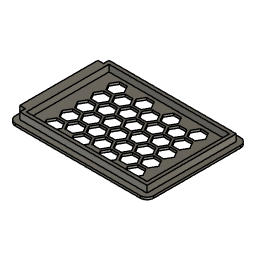
Mini-Amp Case V3 - Cover (Autodesk Fusion 360 design; units mm, degrees)
Autodesk Fusion 360 part; units mm, degrees
(part 1 of 2)
sketch "Sketch1" plane through (0, 0, 0) normal (0, 0, 1) x (1, 0, 0)
  line L0 (-1, -1) -> (57, -1)
  line L1 (57, -1) -> (57, 40)
  line L2 (57, 40) -> (-1, 40)
  line L3 (-1, 40) -> (-1, -1)
  line L4 (-3, -3) -> (59, -3)
  line L5 (59, -3) -> (59, 42)
  line L6 (59, 42) -> (-3, 42)
  line L7 (-3, 42) -> (-3, -3)
  constraint horizontal L0
  constraint vertical L1
  constraint horizontal L2
  constraint vertical L3
  constraint horizontal L4
  constraint vertical L5
  constraint horizontal L6
  constraint vertical L7
extrude "Extrude1" add sketch "Sketch1" along normal blind 3 contours L0 L1 L2 L3 | L4 L5 L6 L7
extrude "Extrude2" add sketch "Sketch1" along normal blind 21
sketch "Sketch2" plane through (59, 0, 0) normal (1, 0, 0) x (0, 1, 0)
  line L0 (-3, 0) -> (42, 0)
  line L1 (42, 0) -> (42, 21)
  line L2 (42, 21) -> (-3, 21)
  line L3 (-3, 21) -> (-3, 0)
  line L4 (42, 0) -> (42, 12.5) construction
  line L5 (42, 12.5) -> (27, 12.5) construction
  circle A0 centre (27, 12.5) radius 5
  dimension "d11" = 15
  dimension "d20" = 12.5
  constraint coincident L0.end L1.start
  constraint coincident L1 L4.end
  constraint perpendicular L0 L4
  constraint perpendicular L4 L5
  constraint coincident L5.end A0.centre
  measures "d11" distance of L1 L5.end
  measures "d20" distance of L0 L5.end
extrude "Extrude3" cut sketch "Sketch2" against normal blind 3 contours A0
sketch "Sketch3" plane through (-3, 0, 0) normal (-1, 0, 0) x (0, -1, 0)
  line L0 (-42, 0) -> (3, 0)
  line L1 (3, 0) -> (3, 21)
  line L2 (3, 21) -> (-42, 21)
  line L3 (-42, 21) -> (-42, 0)
  line L4 (-37, 7) -> (-37, 21)
  line L5 (-37, 21) -> (-2, 21)
  line L6 (-2, 21) -> (-2, 7)
  line L7 (-2, 7) -> (-37, 7)
  constraint perpendicular L0 L4
  constraint perpendicular L1 L5
  constraint perpendicular L5 L6
  constraint perpendicular L4 L7
  constraint coincident L2 L4.end
extrude "Extrude4" cut sketch "Sketch3" against normal blind 3 contours L2 L4 L5 L6 L7
fillet "Fillet1" radius 3 4 edges at (59, -3, 10.5) (59, 42, 10.5) (-3, 42, 10.5) (-3, -3, 10.5)
sketch "Sketch4" plane through (0, 0, 3) normal (0, 0, 1) x (-1, 0, 0)
  line L0 (1, 1) -> (-57, 1)
  line L1 (-57, 1) -> (-57, -40)
  line L2 (-57, -40) -> (1, -40)
  line L3 (1, -40) -> (1, 1)
  point P0 (-29.8405, -19.6761)
extrude "Extrude5" cut 1 faces at (37.3333, 12, 0) along direction (0, 0, 1) blind 1
sketch "Sketch5" plane through (0, 0, 3) normal (0, 0, 1) x (-1, 0, 0)
  line L0 (-8.2346, 0) -> (-7.3686, -1.5)
  line L1 (-7.3686, -1.5) -> (-5.0592, -1.5)
  line L2 (-5.0592, -1.5) -> (-4.1932, 0)
  line L3 (-0.7291, 0) -> (-3.0385, 0)
  line L4 (-3.0385, 0) -> (-4.1932, -2)
  line L5 (-4.1932, -2) -> (-3.0385, -4)
  line L6 (-3.0385, -4) -> (-0.7291, -4)
  line L7 (-0.7291, -4) -> (0, -2.7372)
  line L8 (0, -1.2628) -> (-0.7291, 0)
  line L9 (-16.8949, 0) -> (-16.0289, -1.5)
  line L10 (-16.0289, -1.5) -> (-13.7195, -1.5)
  line L11 (-13.7195, -1.5) -> (-12.8534, 0)
  line L12 (-9.3893, 0) -> (-11.6987, 0)
  line L13 (-11.6987, 0) -> (-12.8534, -2)
  line L14 (-12.8534, -2) -> (-11.6987, -4)
  line L15 (-11.6987, -4) -> (-9.3893, -4)
  line L16 (-9.3893, -4) -> (-8.2346, -2)
  line L17 (-8.2346, -2) -> (-9.3893, 0)
  line L18 (-5.0592, -2.5) -> (-7.3686, -2.5)
  line L19 (-7.3686, -2.5) -> (-8.5233, -4.5)
  line L20 (-8.5233, -4.5) -> (-7.3686, -6.5)
  line L21 (-7.3686, -6.5) -> (-5.0592, -6.5)
  line L22 (-5.0592, -6.5) -> (-3.9045, -4.5)
  line L23 (-3.9045, -4.5) -> (-5.0592, -2.5)
  line L24 (-0.7291, -5) -> (-3.0385, -5)
  line L25 (-3.0385, -5) -> (-4.1932, -7)
  line L26 (-4.1932, -7) -> (-3.0385, -9)
  line L27 (-3.0385, -9) -> (-0.7291, -9)
  line L28 (-0.7291, -9) -> (0, -7.7372)
  line L29 (0, -6.2628) -> (-0.7291, -5)
  line L30 (-25.5551, 0) -> (-24.6891, -1.5)
  line L31 (-24.6891, -1.5) -> (-22.3797, -1.5)
  line L32 (-22.3797, -1.5) -> (-21.5137, 0)
  line L33 (-18.0496, 0) -> (-20.359, 0)
  line L34 (-20.359, 0) -> (-21.5137, -2)
  line L35 (-21.5137, -2) -> (-20.359, -4)
  line L36 (-20.359, -4) -> (-18.0496, -4)
  line L37 (-18.0496, -4) -> (-16.8949, -2)
  line L38 (-16.8949, -2) -> (-18.0496, 0)
  line L39 (-13.7195, -2.5) -> (-16.0289, -2.5)
  line L40 (-16.0289, -2.5) -> (-17.1836, -4.5)
  line L41 (-17.1836, -4.5) -> (-16.0289, -6.5)
  line L42 (-16.0289, -6.5) -> (-13.7195, -6.5)
  line L43 (-13.7195, -6.5) -> (-12.5648, -4.5)
  line L44 (-12.5648, -4.5) -> (-13.7195, -2.5)
  line L45 (-9.3893, -5) -> (-11.6987, -5)
  line L46 (-11.6987, -5) -> (-12.8534, -7)
  line L47 (-12.8534, -7) -> (-11.6987, -9)
  line L48 (-11.6987, -9) -> (-9.3893, -9)
  line L49 (-9.3893, -9) -> (-8.2346, -7)
  line L50 (-8.2346, -7) -> (-9.3893, -5)
  line L51 (-5.0592, -7.5) -> (-7.3686, -7.5)
  line L52 (-7.3686, -7.5) -> (-8.5233, -9.5)
  line L53 (-8.5233, -9.5) -> (-7.3686, -11.5)
  line L54 (-7.3686, -11.5) -> (-5.0592, -11.5)
  line L55 (-5.0592, -11.5) -> (-3.9045, -9.5)
  line L56 (-3.9045, -9.5) -> (-5.0592, -7.5)
  line L57 (-0.7291, -10) -> (-3.0385, -10)
  line L58 (-3.0385, -10) -> (-4.1932, -12)
  line L59 (-4.1932, -12) -> (-3.0385, -14)
  line L60 (-3.0385, -14) -> (-0.7291, -14)
  line L61 (-0.7291, -14) -> (0, -12.7372)
  line L62 (0, -11.2628) -> (-0.7291, -10)
  line L63 (-34.2154, 0) -> (-33.3494, -1.5)
  line L64 (-33.3494, -1.5) -> (-31.04, -1.5)
  line L65 (-31.04, -1.5) -> (-30.1739, 0)
  line L66 (-26.7098, 0) -> (-29.0192, 0)
  line L67 (-29.0192, 0) -> (-30.1739, -2)
  line L68 (-30.1739, -2) -> (-29.0192, -4)
  line L69 (-29.0192, -4) -> (-26.7098, -4)
  line L70 (-26.7098, -4) -> (-25.5551, -2)
  line L71 (-25.5551, -2) -> (-26.7098, 0)
  line L72 (-22.3797, -2.5) -> (-24.6891, -2.5)
  line L73 (-24.6891, -2.5) -> (-25.8438, -4.5)
  line L74 (-25.8438, -4.5) -> (-24.6891, -6.5)
  line L75 (-24.6891, -6.5) -> (-22.3797, -6.5)
  line L76 (-22.3797, -6.5) -> (-21.225, -4.5)
  line L77 (-21.225, -4.5) -> (-22.3797, -2.5)
  line L78 (-18.0496, -5) -> (-20.359, -5)
  line L79 (-20.359, -5) -> (-21.5137, -7)
  line L80 (-21.5137, -7) -> (-20.359, -9)
  line L81 (-20.359, -9) -> (-18.0496, -9)
  line L82 (-18.0496, -9) -> (-16.8949, -7)
  line L83 (-16.8949, -7) -> (-18.0496, -5)
  line L84 (-13.7195, -7.5) -> (-16.0289, -7.5)
  line L85 (-16.0289, -7.5) -> (-17.1836, -9.5)
  line L86 (-17.1836, -9.5) -> (-16.0289, -11.5)
  line L87 (-16.0289, -11.5) -> (-13.7195, -11.5)
  line L88 (-13.7195, -11.5) -> (-12.5648, -9.5)
  line L89 (-12.5648, -9.5) -> (-13.7195, -7.5)
  line L90 (-9.3893, -10) -> (-11.6987, -10)
  line L91 (-11.6987, -10) -> (-12.8534, -12)
  line L92 (-12.8534, -12) -> (-11.6987, -14)
  line L93 (-11.6987, -14) -> (-9.3893, -14)
  line L94 (-9.3893, -14) -> (-8.2346, -12)
  line L95 (-8.2346, -12) -> (-9.3893, -10)
  line L96 (-5.0592, -12.5) -> (-7.3686, -12.5)
  line L97 (-7.3686, -12.5) -> (-8.5233, -14.5)
  line L98 (-8.5233, -14.5) -> (-7.3686, -16.5)
  line L99 (-7.3686, -16.5) -> (-5.0592, -16.5)
  line L100 (-5.0592, -16.5) -> (-3.9045, -14.5)
  line L101 (-3.9045, -14.5) -> (-5.0592, -12.5)
  line L102 (-0.7291, -15) -> (-3.0385, -15)
  line L103 (-3.0385, -15) -> (-4.1932, -17)
  line L104 (-4.1932, -17) -> (-3.0385, -19)
  line L105 (-3.0385, -19) -> (-0.7291, -19)
  line L106 (-0.7291, -19) -> (0, -17.7372)
  line L107 (0, -16.2628) -> (-0.7291, -15)
  line L108 (-42.8756, 0) -> (-42.0096, -1.5)
  line L109 (-42.0096, -1.5) -> (-39.7002, -1.5)
  line L110 (-39.7002, -1.5) -> (-38.8342, 0)
  line L111 (-35.3701, 0) -> (-37.6795, 0)
  line L112 (-37.6795, 0) -> (-38.8342, -2)
  line L113 (-38.8342, -2) -> (-37.6795, -4)
  line L114 (-37.6795, -4) -> (-35.3701, -4)
  line L115 (-35.3701, -4) -> (-34.2154, -2)
  line L116 (-34.2154, -2) -> (-35.3701, 0)
  line L117 (-31.04, -2.5) -> (-33.3494, -2.5)
  line L118 (-33.3494, -2.5) -> (-34.5041, -4.5)
  line L119 (-34.5041, -4.5) -> (-33.3494, -6.5)
  line L120 (-33.3494, -6.5) -> (-31.04, -6.5)
  line L121 (-31.04, -6.5) -> (-29.8853, -4.5)
  line L122 (-29.8853, -4.5) -> (-31.04, -2.5)
  line L123 (-26.7098, -5) -> (-29.0192, -5)
  line L124 (-29.0192, -5) -> (-30.1739, -7)
  line L125 (-30.1739, -7) -> (-29.0192, -9)
  line L126 (-29.0192, -9) -> (-26.7098, -9)
  line L127 (-26.7098, -9) -> (-25.5551, -7)
  line L128 (-25.5551, -7) -> (-26.7098, -5)
  line L129 (-22.3797, -7.5) -> (-24.6891, -7.5)
  line L130 (-24.6891, -7.5) -> (-25.8438, -9.5)
  line L131 (-25.8438, -9.5) -> (-24.6891, -11.5)
  line L132 (-24.6891, -11.5) -> (-22.3797, -11.5)
  line L133 (-22.3797, -11.5) -> (-21.225, -9.5)
  line L134 (-21.225, -9.5) -> (-22.3797, -7.5)
  line L135 (-18.0496, -10) -> (-20.359, -10)
  line L136 (-20.359, -10) -> (-21.5137, -12)
  line L137 (-21.5137, -12) -> (-20.359, -14)
  line L138 (-20.359, -14) -> (-18.0496, -14)
  line L139 (-18.0496, -14) -> (-16.8949, -12)
  line L140 (-16.8949, -12) -> (-18.0496, -10)
  line L141 (-13.7195, -12.5) -> (-16.0289, -12.5)
  line L142 (-16.0289, -12.5) -> (-17.1836, -14.5)
  line L143 (-17.1836, -14.5) -> (-16.0289, -16.5)
  line L144 (-16.0289, -16.5) -> (-13.7195, -16.5)
  line L145 (-13.7195, -16.5) -> (-12.5648, -14.5)
  line L146 (-12.5648, -14.5) -> (-13.7195, -12.5)
  line L147 (-9.3893, -15) -> (-11.6987, -15)
  line L148 (-11.6987, -15) -> (-12.8534, -17)
  line L149 (-12.8534, -17) -> (-11.6987, -19)
  line L150 (-11.6987, -19) -> (-9.3893, -19)
  line L151 (-9.3893, -19) -> (-8.2346, -17)
  line L152 (-8.2346, -17) -> (-9.3893, -15)
  line L153 (-5.0592, -17.5) -> (-7.3686, -17.5)
  line L154 (-7.3686, -17.5) -> (-8.5233, -19.5)
  line L155 (-8.5233, -19.5) -> (-7.3686, -21.5)
  line L156 (-7.3686, -21.5) -> (-5.0592, -21.5)
  line L157 (-5.0592, -21.5) -> (-3.9045, -19.5)
  line L158 (-3.9045, -19.5) -> (-5.0592, -17.5)
  line L159 (-0.7291, -20) -> (-3.0385, -20)
  line L160 (-3.0385, -20) -> (-4.1932, -22)
  line L161 (-4.1932, -22) -> (-3.0385, -24)
  line L162 (-3.0385, -24) -> (-0.7291, -24)
  line L163 (-0.7291, -24) -> (0, -22.7372)
  line L164 (0, -21.2628) -> (-0.7291, -20)
  line L165 (-51.5359, 0) -> (-50.6699, -1.5)
  line L166 (-50.6699, -1.5) -> (-48.3605, -1.5)
  line L167 (-48.3605, -1.5) -> (-47.4944, 0)
  line L168 (-44.0303, 0) -> (-46.3397, 0)
  line L169 (-46.3397, 0) -> (-47.4944, -2)
  line L170 (-47.4944, -2) -> (-46.3397, -4)
  line L171 (-46.3397, -4) -> (-44.0303, -4)
  line L172 (-44.0303, -4) -> (-42.8756, -2)
  line L173 (-42.8756, -2) -> (-44.0303, 0)
  line L174 (-39.7002, -2.5) -> (-42.0096, -2.5)
  line L175 (-42.0096, -2.5) -> (-43.1643, -4.5)
  line L176 (-43.1643, -4.5) -> (-42.0096, -6.5)
  line L177 (-42.0096, -6.5) -> (-39.7002, -6.5)
  line L178 (-39.7002, -6.5) -> (-38.5455, -4.5)
  line L179 (-38.5455, -4.5) -> (-39.7002, -2.5)
  line L180 (-35.3701, -5) -> (-37.6795, -5)
  line L181 (-37.6795, -5) -> (-38.8342, -7)
  line L182 (-38.8342, -7) -> (-37.6795, -9)
  line L183 (-37.6795, -9) -> (-35.3701, -9)
  line L184 (-35.3701, -9) -> (-34.2154, -7)
  line L185 (-34.2154, -7) -> (-35.3701, -5)
  line L186 (-31.04, -7.5) -> (-33.3494, -7.5)
  line L187 (-33.3494, -7.5) -> (-34.5041, -9.5)
  line L188 (-34.5041, -9.5) -> (-33.3494, -11.5)
  line L189 (-33.3494, -11.5) -> (-31.04, -11.5)
  line L190 (-31.04, -11.5) -> (-29.8853, -9.5)
  line L191 (-29.8853, -9.5) -> (-31.04, -7.5)
  line L192 (-26.7098, -10) -> (-29.0192, -10)
  line L193 (-29.0192, -10) -> (-30.1739, -12)
  line L194 (-30.1739, -12) -> (-29.0192, -14)
  line L195 (-29.0192, -14) -> (-26.7098, -14)
  line L196 (-26.7098, -14) -> (-25.5551, -12)
  line L197 (-25.5551, -12) -> (-26.7098, -10)
  line L198 (-22.3797, -12.5) -> (-24.6891, -12.5)
  line L199 (-24.6891, -12.5) -> (-25.8438, -14.5)
  line L200 (-25.8438, -14.5) -> (-24.6891, -16.5)
  line L201 (-24.6891, -16.5) -> (-22.3797, -16.5)
  line L202 (-22.3797, -16.5) -> (-21.225, -14.5)
  line L203 (-21.225, -14.5) -> (-22.3797, -12.5)
  line L204 (-18.0496, -15) -> (-20.359, -15)
  line L205 (-20.359, -15) -> (-21.5137, -17)
  line L206 (-21.5137, -17) -> (-20.359, -19)
  line L207 (-20.359, -19) -> (-18.0496, -19)
  line L208 (-18.0496, -19) -> (-16.8949, -17)
  line L209 (-16.8949, -17) -> (-18.0496, -15)
  line L210 (-13.7195, -17.5) -> (-16.0289, -17.5)
  line L211 (-16.0289, -17.5) -> (-17.1836, -19.5)
  line L212 (-17.1836, -19.5) -> (-16.0289, -21.5)
  line L213 (-16.0289, -21.5) -> (-13.7195, -21.5)
  line L214 (-13.7195, -21.5) -> (-12.5648, -19.5)
  line L215 (-12.5648, -19.5) -> (-13.7195, -17.5)
  line L216 (-9.3893, -20) -> (-11.6987, -20)
  line L217 (-11.6987, -20) -> (-12.8534, -22)
  line L218 (-12.8534, -22) -> (-11.6987, -24)
  line L219 (-11.6987, -24) -> (-9.3893, -24)
  line L220 (-9.3893, -24) -> (-8.2346, -22)
  line L221 (-8.2346, -22) -> (-9.3893, -20)
  line L222 (-5.0592, -22.5) -> (-7.3686, -22.5)
  line L223 (-7.3686, -22.5) -> (-8.5233, -24.5)
  line L224 (-8.5233, -24.5) -> (-7.3686, -26.5)
  line L225 (-7.3686, -26.5) -> (-5.0592, -26.5)
  line L226 (-5.0592, -26.5) -> (-3.9045, -24.5)
  line L227 (-3.9045, -24.5) -> (-5.0592, -22.5)
  line L228 (-0.7291, -25) -> (-3.0385, -25)
  line L229 (-3.0385, -25) -> (-4.1932, -27)
  line L230 (-4.1932, -27) -> (-3.0385, -29)
  line L231 (-3.0385, -29) -> (-0.7291, -29)
  line L232 (-0.7291, -29) -> (0, -27.7372)
  line L233 (0, -26.2628) -> (-0.7291, -25)
  line L234 (-52.6906, 0) -> (-55, 0)
  line L235 (-55, 0) -> (-56, -1.7321)
  line L236 (-56, -2.2679) -> (-55, -4)
  line L237 (-55, -4) -> (-52.6906, -4)
  line L238 (-52.6906, -4) -> (-51.5359, -2)
  line L239 (-51.5359, -2) -> (-52.6906, 0)
  line L240 (-48.3605, -2.5) -> (-50.6699, -2.5)
  line L241 (-50.6699, -2.5) -> (-51.8246, -4.5)
  line L242 (-51.8246, -4.5) -> (-50.6699, -6.5)
  line L243 (-50.6699, -6.5) -> (-48.3605, -6.5)
  line L244 (-48.3605, -6.5) -> (-47.2058, -4.5)
  line L245 (-47.2058, -4.5) -> (-48.3605, -2.5)
  line L246 (-44.0303, -5) -> (-46.3397, -5)
  line L247 (-46.3397, -5) -> (-47.4944, -7)
  line L248 (-47.4944, -7) -> (-46.3397, -9)
  line L249 (-46.3397, -9) -> (-44.0303, -9)
  line L250 (-44.0303, -9) -> (-42.8756, -7)
  line L251 (-42.8756, -7) -> (-44.0303, -5)
  line L252 (-39.7002, -7.5) -> (-42.0096, -7.5)
  line L253 (-42.0096, -7.5) -> (-43.1643, -9.5)
  line L254 (-43.1643, -9.5) -> (-42.0096, -11.5)
  line L255 (-42.0096, -11.5) -> (-39.7002, -11.5)
  line L256 (-39.7002, -11.5) -> (-38.5455, -9.5)
  line L257 (-38.5455, -9.5) -> (-39.7002, -7.5)
  line L258 (-35.3701, -10) -> (-37.6795, -10)
  line L259 (-37.6795, -10) -> (-38.8342, -12)
  line L260 (-38.8342, -12) -> (-37.6795, -14)
  line L261 (-37.6795, -14) -> (-35.3701, -14)
  line L262 (-35.3701, -14) -> (-34.2154, -12)
  line L263 (-34.2154, -12) -> (-35.3701, -10)
  line L264 (-31.04, -12.5) -> (-33.3494, -12.5)
  line L265 (-33.3494, -12.5) -> (-34.5041, -14.5)
  line L266 (-34.5041, -14.5) -> (-33.3494, -16.5)
  line L267 (-33.3494, -16.5) -> (-31.04, -16.5)
  line L268 (-31.04, -16.5) -> (-29.8853, -14.5)
  line L269 (-29.8853, -14.5) -> (-31.04, -12.5)
  line L270 (-26.7098, -15) -> (-29.0192, -15)
  line L271 (-29.0192, -15) -> (-30.1739, -17)
  line L272 (-30.1739, -17) -> (-29.0192, -19)
  line L273 (-29.0192, -19) -> (-26.7098, -19)
  line L274 (-26.7098, -19) -> (-25.5551, -17)
  line L275 (-25.5551, -17) -> (-26.7098, -15)
  line L276 (-22.3797, -17.5) -> (-24.6891, -17.5)
  line L277 (-24.6891, -17.5) -> (-25.8438, -19.5)
  line L278 (-25.8438, -19.5) -> (-24.6891, -21.5)
  line L279 (-24.6891, -21.5) -> (-22.3797, -21.5)
  line L280 (-22.3797, -21.5) -> (-21.225, -19.5)
  line L281 (-21.225, -19.5) -> (-22.3797, -17.5)
  line L282 (-18.0496, -20) -> (-20.359, -20)
  line L283 (-20.359, -20) -> (-21.5137, -22)
  line L284 (-21.5137, -22) -> (-20.359, -24)
  line L285 (-20.359, -24) -> (-18.0496, -24)
  line L286 (-18.0496, -24) -> (-16.8949, -22)
  line L287 (-16.8949, -22) -> (-18.0496, -20)
  line L288 (-13.7195, -22.5) -> (-16.0289, -22.5)
  line L289 (-16.0289, -22.5) -> (-17.1836, -24.5)
  line L290 (-17.1836, -24.5) -> (-16.0289, -26.5)
  line L291 (-16.0289, -26.5) -> (-13.7195, -26.5)
  line L292 (-13.7195, -26.5) -> (-12.5648, -24.5)
  line L293 (-12.5648, -24.5) -> (-13.7195, -22.5)
  line L294 (-9.3893, -25) -> (-11.6987, -25)
  line L295 (-11.6987, -25) -> (-12.8534, -27)
  line L296 (-12.8534, -27) -> (-11.6987, -29)
  line L297 (-11.6987, -29) -> (-9.3893, -29)
  line L298 (-9.3893, -29) -> (-8.2346, -27)
  line L299 (-8.2346, -27) -> (-9.3893, -25)
  line L300 (-5.0592, -27.5) -> (-7.3686, -27.5)
  line L301 (-7.3686, -27.5) -> (-8.5233, -29.5)
  line L302 (-8.5233, -29.5) -> (-7.3686, -31.5)
  line L303 (-7.3686, -31.5) -> (-5.0592, -31.5)
  line L304 (-5.0592, -31.5) -> (-3.9045, -29.5)
  line L305 (-3.9045, -29.5) -> (-5.0592, -27.5)
  line L306 (-0.7291, -30) -> (-3.0385, -30)
  line L307 (-3.0385, -30) -> (-4.1932, -32)
  line L308 (-4.1932, -32) -> (-3.0385, -34)
  line L309 (-3.0385, -34) -> (-0.7291, -34)
  line L310 (-0.7291, -34) -> (0, -32.7372)
  line L311 (0, -31.2628) -> (-0.7291, -30)
  line L312 (-52.6906, -5) -> (-55, -5)
  line L313 (-55, -5) -> (-56, -6.7321)
  line L314 (-56, -7.2679) -> (-55, -9)
  line L315 (-55, -9) -> (-52.6906, -9)
  line L316 (-52.6906, -9) -> (-51.5359, -7)
  line L317 (-51.5359, -7) -> (-52.6906, -5)
  line L318 (-48.3605, -7.5) -> (-50.6699, -7.5)
  line L319 (-50.6699, -7.5) -> (-51.8246, -9.5)
  line L320 (-51.8246, -9.5) -> (-50.6699, -11.5)
  line L321 (-50.6699, -11.5) -> (-48.3605, -11.5)
  line L322 (-48.3605, -11.5) -> (-47.2058, -9.5)
  line L323 (-47.2058, -9.5) -> (-48.3605, -7.5)
  line L324 (-44.0303, -10) -> (-46.3397, -10)
  line L325 (-46.3397, -10) -> (-47.4944, -12)
  line L326 (-47.4944, -12) -> (-46.3397, -14)
  line L327 (-46.3397, -14) -> (-44.0303, -14)
  line L328 (-44.0303, -14) -> (-42.8756, -12)
  line L329 (-42.8756, -12) -> (-44.0303, -10)
  line L330 (-39.7002, -12.5) -> (-42.0096, -12.5)
  line L331 (-42.0096, -12.5) -> (-43.1643, -14.5)
  line L332 (-43.1643, -14.5) -> (-42.0096, -16.5)
  line L333 (-42.0096, -16.5) -> (-39.7002, -16.5)
  line L334 (-39.7002, -16.5) -> (-38.5455, -14.5)
  line L335 (-38.5455, -14.5) -> (-39.7002, -12.5)
  line L336 (-35.3701, -15) -> (-37.6795, -15)
  line L337 (-37.6795, -15) -> (-38.8342, -17)
  line L338 (-38.8342, -17) -> (-37.6795, -19)
  line L339 (-37.6795, -19) -> (-35.3701, -19)
  line L340 (-35.3701, -19) -> (-34.2154, -17)
  line L341 (-34.2154, -17) -> (-35.3701, -15)
  line L342 (-31.04, -17.5) -> (-33.3494, -17.5)
  line L343 (-33.3494, -17.5) -> (-34.5041, -19.5)
  line L344 (-34.5041, -19.5) -> (-33.3494, -21.5)
  line L345 (-33.3494, -21.5) -> (-31.04, -21.5)
  line L346 (-31.04, -21.5) -> (-29.8853, -19.5)
  line L347 (-29.8853, -19.5) -> (-31.04, -17.5)
  line L348 (-26.7098, -20) -> (-29.0192, -20)
  line L349 (-29.0192, -20) -> (-30.1739, -22)
  line L350 (-30.1739, -22) -> (-29.0192, -24)
  line L351 (-29.0192, -24) -> (-26.7098, -24)
  line L352 (-26.7098, -24) -> (-25.5551, -22)
  line L353 (-25.5551, -22) -> (-26.7098, -20)
  line L354 (-22.3797, -22.5) -> (-24.6891, -22.5)
  line L355 (-24.6891, -22.5) -> (-25.8438, -24.5)
  line L356 (-25.8438, -24.5) -> (-24.6891, -26.5)
  line L357 (-24.6891, -26.5) -> (-22.3797, -26.5)
  line L358 (-22.3797, -26.5) -> (-21.225, -24.5)
  line L359 (-21.225, -24.5) -> (-22.3797, -22.5)
  line L360 (-18.0496, -25) -> (-20.359, -25)
  line L361 (-20.359, -25) -> (-21.5137, -27)
  line L362 (-21.5137, -27) -> (-20.359, -29)
  line L363 (-20.359, -29) -> (-18.0496, -29)
  line L364 (-18.0496, -29) -> (-16.8949, -27)
  line L365 (-16.8949, -27) -> (-18.0496, -25)
  line L366 (-13.7195, -27.5) -> (-16.0289, -27.5)
  line L367 (-16.0289, -27.5) -> (-17.1836, -29.5)
  line L368 (-17.1836, -29.5) -> (-16.0289, -31.5)
  line L369 (-16.0289, -31.5) -> (-13.7195, -31.5)
  line L370 (-13.7195, -31.5) -> (-12.5648, -29.5)
  line L371 (-12.5648, -29.5) -> (-13.7195, -27.5)
  line L372 (-9.3893, -30) -> (-11.6987, -30)
  line L373 (-11.6987, -30) -> (-12.8534, -32)
  line L374 (-12.8534, -32) -> (-11.6987, -34)
  line L375 (-11.6987, -34) -> (-9.3893, -34)
  line L376 (-9.3893, -34) -> (-8.2346, -32)
  line L377 (-8.2346, -32) -> (-9.3893, -30)
  line L378 (-5.0592, -32.5) -> (-7.3686, -32.5)
  line L379 (-7.3686, -32.5) -> (-8.5233, -34.5)
  line L380 (-8.5233, -34.5) -> (-7.3686, -36.5)
  line L381 (-7.3686, -36.5) -> (-5.0592, -36.5)
  line L382 (-5.0592, -36.5) -> (-3.9045, -34.5)
  line L383 (-3.9045, -34.5) -> (-5.0592, -32.5)
  line L384 (-0.7291, -35) -> (-3.0385, -35)
  line L385 (-3.0385, -35) -> (-4.1932, -37)
  line L386 (-4.1932, -37) -> (-3.0385, -39)
  line L387 (-3.0385, -39) -> (-0.7291, -39)
  line L388 (-0.7291, -39) -> (0, -37.7372)
  line L389 (0, -36.2628) -> (-0.7291, -35)
  line L390 (-52.6906, -10) -> (-55, -10)
  line L391 (-55, -10) -> (-56, -11.7321)
  line L392 (-56, -12.2679) -> (-55, -14)
  line L393 (-55, -14) -> (-52.6906, -14)
  line L394 (-52.6906, -14) -> (-51.5359, -12)
  line L395 (-51.5359, -12) -> (-52.6906, -10)
  line L396 (-48.3605, -12.5) -> (-50.6699, -12.5)
  line L397 (-50.6699, -12.5) -> (-51.8246, -14.5)
  line L398 (-51.8246, -14.5) -> (-50.6699, -16.5)
  line L399 (-50.6699, -16.5) -> (-48.3605, -16.5)
  line L400 (-48.3605, -16.5) -> (-47.2058, -14.5)
  line L401 (-47.2058, -14.5) -> (-48.3605, -12.5)
  line L402 (-44.0303, -15) -> (-46.3397, -15)
  line L403 (-46.3397, -15) -> (-47.4944, -17)
  line L404 (-47.4944, -17) -> (-46.3397, -19)
  line L405 (-46.3397, -19) -> (-44.0303, -19)
  line L406 (-44.0303, -19) -> (-42.8756, -17)
  line L407 (-42.8756, -17) -> (-44.0303, -15)
  line L408 (-39.7002, -17.5) -> (-42.0096, -17.5)
  line L409 (-42.0096, -17.5) -> (-43.1643, -19.5)
  line L410 (-43.1643, -19.5) -> (-42.0096, -21.5)
  line L411 (-42.0096, -21.5) -> (-39.7002, -21.5)
  line L412 (-39.7002, -21.5) -> (-38.5455, -19.5)
  line L413 (-38.5455, -19.5) -> (-39.7002, -17.5)
  line L414 (-35.3701, -20) -> (-37.6795, -20)
  line L415 (-37.6795, -20) -> (-38.8342, -22)
  line L416 (-38.8342, -22) -> (-37.6795, -24)
  line L417 (-37.6795, -24) -> (-35.3701, -24)
  line L418 (-35.3701, -24) -> (-34.2154, -22)
  line L419 (-34.2154, -22) -> (-35.3701, -20)
  line L420 (-31.04, -22.5) -> (-33.3494, -22.5)
  line L421 (-33.3494, -22.5) -> (-34.5041, -24.5)
  line L422 (-34.5041, -24.5) -> (-33.3494, -26.5)
  line L423 (-33.3494, -26.5) -> (-31.04, -26.5)
  line L424 (-31.04, -26.5) -> (-29.8853, -24.5)
  line L425 (-29.8853, -24.5) -> (-31.04, -22.5)
  line L426 (-26.7098, -25) -> (-29.0192, -25)
  line L427 (-29.0192, -25) -> (-30.1739, -27)
  line L428 (-30.1739, -27) -> (-29.0192, -29)
  line L429 (-29.0192, -29) -> (-26.7098, -29)
  line L430 (-26.7098, -29) -> (-25.5551, -27)
  line L431 (-25.5551, -27) -> (-26.7098, -25)
  line L432 (-22.3797, -27.5) -> (-24.6891, -27.5)
  line L433 (-24.6891, -27.5) -> (-25.8438, -29.5)
  line L434 (-25.8438, -29.5) -> (-24.6891, -31.5)
  line L435 (-24.6891, -31.5) -> (-22.3797, -31.5)
  line L436 (-22.3797, -31.5) -> (-21.225, -29.5)
  line L437 (-21.225, -29.5) -> (-22.3797, -27.5)
  line L438 (-18.0496, -30) -> (-20.359, -30)
  line L439 (-20.359, -30) -> (-21.5137, -32)
  line L440 (-21.5137, -32) -> (-20.359, -34)
  line L441 (-20.359, -34) -> (-18.0496, -34)
  line L442 (-18.0496, -34) -> (-16.8949, -32)
  line L443 (-16.8949, -32) -> (-18.0496, -30)
  line L444 (-13.7195, -32.5) -> (-16.0289, -32.5)
  line L445 (-16.0289, -32.5) -> (-17.1836, -34.5)
  line L446 (-17.1836, -34.5) -> (-16.0289, -36.5)
  line L447 (-16.0289, -36.5) -> (-13.7195, -36.5)
  line L448 (-13.7195, -36.5) -> (-12.5648, -34.5)
  line L449 (-12.5648, -34.5) -> (-13.7195, -32.5)
  line L450 (-9.3893, -35) -> (-11.6987, -35)
  line L451 (-11.6987, -35) -> (-12.8534, -37)
  line L452 (-12.8534, -37) -> (-11.6987, -39)
  line L453 (-11.6987, -39) -> (-9.3893, -39)
  line L454 (-9.3893, -39) -> (-8.2346, -37)
  line L455 (-8.2346, -37) -> (-9.3893, -35)
  line L456 (-5.0592, -37.5) -> (-7.3686, -37.5)
  line L457 (-7.3686, -37.5) -> (-8.2346, -39)
  line L458 (-4.1932, -39) -> (-5.0592, -37.5)
  line L459 (-52.6906, -15) -> (-55, -15)
  line L460 (-55, -15) -> (-56, -16.7321)
  line L461 (-56, -17.2679) -> (-55, -19)
  line L462 (-55, -19) -> (-52.6906, -19)
  line L463 (-52.6906, -19) -> (-51.5359, -17)
  line L464 (-51.5359, -17) -> (-52.6906, -15)
  line L465 (-48.3605, -17.5) -> (-50.6699, -17.5)
  line L466 (-50.6699, -17.5) -> (-51.8246, -19.5)
  line L467 (-51.8246, -19.5) -> (-50.6699, -21.5)
  line L468 (-50.6699, -21.5) -> (-48.3605, -21.5)
  line L469 (-48.3605, -21.5) -> (-47.2058, -19.5)
  line L470 (-47.2058, -19.5) -> (-48.3605, -17.5)
  line L471 (-44.0303, -20) -> (-46.3397, -20)
  line L472 (-46.3397, -20) -> (-47.4944, -22)
  line L473 (-47.4944, -22) -> (-46.3397, -24)
  line L474 (-46.3397, -24) -> (-44.0303, -24)
  line L475 (-44.0303, -24) -> (-42.8756, -22)
  line L476 (-42.8756, -22) -> (-44.0303, -20)
  line L477 (-39.7002, -22.5) -> (-42.0096, -22.5)
  line L478 (-42.0096, -22.5) -> (-43.1643, -24.5)
  line L479 (-43.1643, -24.5) -> (-42.0096, -26.5)
  line L480 (-42.0096, -26.5) -> (-39.7002, -26.5)
  line L481 (-39.7002, -26.5) -> (-38.5455, -24.5)
  line L482 (-38.5455, -24.5) -> (-39.7002, -22.5)
  line L483 (-35.3701, -25) -> (-37.6795, -25)
  line L484 (-37.6795, -25) -> (-38.8342, -27)
  line L485 (-38.8342, -27) -> (-37.6795, -29)
  line L486 (-37.6795, -29) -> (-35.3701, -29)
  line L487 (-35.3701, -29) -> (-34.2154, -27)
  line L488 (-34.2154, -27) -> (-35.3701, -25)
  line L489 (-31.04, -27.5) -> (-33.3494, -27.5)
  line L490 (-33.3494, -27.5) -> (-34.5041, -29.5)
  line L491 (-34.5041, -29.5) -> (-33.3494, -31.5)
  line L492 (-33.3494, -31.5) -> (-31.04, -31.5)
  line L493 (-31.04, -31.5) -> (-29.8853, -29.5)
  line L494 (-29.8853, -29.5) -> (-31.04, -27.5)
  line L495 (-26.7098, -30) -> (-29.0192, -30)
  line L496 (-29.0192, -30) -> (-30.1739, -32)
  line L497 (-30.1739, -32) -> (-29.0192, -34)
  line L498 (-29.0192, -34) -> (-26.7098, -34)
  line L499 (-26.7098, -34) -> (-25.5551, -32)
  line L500 (-25.5551, -32) -> (-26.7098, -30)
  line L501 (-22.3797, -32.5) -> (-24.6891, -32.5)
  line L502 (-24.6891, -32.5) -> (-25.8438, -34.5)
  line L503 (-25.8438, -34.5) -> (-24.6891, -36.5)
  line L504 (-24.6891, -36.5) -> (-22.3797, -36.5)
  line L505 (-22.3797, -36.5) -> (-21.225, -34.5)
  line L506 (-21.225, -34.5) -> (-22.3797, -32.5)
  line L507 (-18.0496, -35) -> (-20.359, -35)
  line L508 (-20.359, -35) -> (-21.5137, -37)
  line L509 (-21.5137, -37) -> (-20.359, -39)
  line L510 (-20.359, -39) -> (-18.0496, -39)
  line L511 (-18.0496, -39) -> (-16.8949, -37)
  line L512 (-16.8949, -37) -> (-18.0496, -35)
  line L513 (-13.7195, -37.5) -> (-16.0289, -37.5)
  line L514 (-16.0289, -37.5) -> (-16.8949, -39)
  line L515 (-12.8534, -39) -> (-13.7195, -37.5)
  line L516 (-52.6906, -20) -> (-55, -20)
  line L517 (-55, -20) -> (-56, -21.7321)
  line L518 (-56, -22.2679) -> (-55, -24)
  line L519 (-55, -24) -> (-52.6906, -24)
  line L520 (-52.6906, -24) -> (-51.5359, -22)
  line L521 (-51.5359, -22) -> (-52.6906, -20)
  line L522 (-48.3605, -22.5) -> (-50.6699, -22.5)
  line L523 (-50.6699, -22.5) -> (-51.8246, -24.5)
  line L524 (-51.8246, -24.5) -> (-50.6699, -26.5)
  line L525 (-50.6699, -26.5) -> (-48.3605, -26.5)
  line L526 (-48.3605, -26.5) -> (-47.2058, -24.5)
  line L527 (-47.2058, -24.5) -> (-48.3605, -22.5)
  line L528 (-44.0303, -25) -> (-46.3397, -25)
  line L529 (-46.3397, -25) -> (-47.4944, -27)
  line L530 (-47.4944, -27) -> (-46.3397, -29)
  line L531 (-46.3397, -29) -> (-44.0303, -29)
  line L532 (-44.0303, -29) -> (-42.8756, -27)
  line L533 (-42.8756, -27) -> (-44.0303, -25)
  line L534 (-39.7002, -27.5) -> (-42.0096, -27.5)
  line L535 (-42.0096, -27.5) -> (-43.1643, -29.5)
  line L536 (-43.1643, -29.5) -> (-42.0096, -31.5)
  line L537 (-42.0096, -31.5) -> (-39.7002, -31.5)
  line L538 (-39.7002, -31.5) -> (-38.5455, -29.5)
  line L539 (-38.5455, -29.5) -> (-39.7002, -27.5)
  line L540 (-35.3701, -30) -> (-37.6795, -30)
  line L541 (-37.6795, -30) -> (-38.8342, -32)
  line L542 (-38.8342, -32) -> (-37.6795, -34)
  line L543 (-37.6795, -34) -> (-35.3701, -34)
  line L544 (-35.3701, -34) -> (-34.2154, -32)
  line L545 (-34.2154, -32) -> (-35.3701, -30)
  line L546 (-31.04, -32.5) -> (-33.3494, -32.5)
  line L547 (-33.3494, -32.5) -> (-34.5041, -34.5)
  line L548 (-34.5041, -34.5) -> (-33.3494, -36.5)
  line L549 (-33.3494, -36.5) -> (-31.04, -36.5)
  line L550 (-31.04, -36.5) -> (-29.8853, -34.5)
  line L551 (-29.8853, -34.5) -> (-31.04, -32.5)
  line L552 (-26.7098, -35) -> (-29.0192, -35)
  line L553 (-29.0192, -35) -> (-30.1739, -37)
  line L554 (-30.1739, -37) -> (-29.0192, -39)
  line L555 (-29.0192, -39) -> (-26.7098, -39)
  line L556 (-26.7098, -39) -> (-25.5551, -37)
  line L557 (-25.5551, -37) -> (-26.7098, -35)
  line L558 (-22.3797, -37.5) -> (-24.6891, -37.5)
  line L559 (-24.6891, -37.5) -> (-25.5551, -39)
  line L560 (-21.5137, -39) -> (-22.3797, -37.5)
  line L561 (-52.6906, -25) -> (-55, -25)
  line L562 (-55, -25) -> (-56, -26.7321)
  line L563 (-56, -27.2679) -> (-55, -29)
  line L564 (-55, -29) -> (-52.6906, -29)
  line L565 (-52.6906, -29) -> (-51.5359, -27)
  line L566 (-51.5359, -27) -> (-52.6906, -25)
  line L567 (-48.3605, -27.5) -> (-50.6699, -27.5)
  line L568 (-50.6699, -27.5) -> (-51.8246, -29.5)
  line L569 (-51.8246, -29.5) -> (-50.6699, -31.5)
  line L570 (-50.6699, -31.5) -> (-48.3605, -31.5)
  line L571 (-48.3605, -31.5) -> (-47.2058, -29.5)
  line L572 (-47.2058, -29.5) -> (-48.3605, -27.5)
  line L573 (-44.0303, -30) -> (-46.3397, -30)
  line L574 (-46.3397, -30) -> (-47.4944, -32)
  line L575 (-47.4944, -32) -> (-46.3397, -34)
  line L576 (-46.3397, -34) -> (-44.0303, -34)
  line L577 (-44.0303, -34) -> (-42.8756, -32)
  line L578 (-42.8756, -32) -> (-44.0303, -30)
  line L579 (-39.7002, -32.5) -> (-42.0096, -32.5)
  line L580 (-42.0096, -32.5) -> (-43.1643, -34.5)
  line L581 (-43.1643, -34.5) -> (-42.0096, -36.5)
  line L582 (-42.0096, -36.5) -> (-39.7002, -36.5)
  line L583 (-39.7002, -36.5) -> (-38.5455, -34.5)
  line L584 (-38.5455, -34.5) -> (-39.7002, -32.5)
  line L585 (-35.3701, -35) -> (-37.6795, -35)
  line L586 (-37.6795, -35) -> (-38.8342, -37)
  line L587 (-38.8342, -37) -> (-37.6795, -39)
  line L588 (-37.6795, -39) -> (-35.3701, -39)
  line L589 (-35.3701, -39) -> (-34.2154, -37)
  line L590 (-34.2154, -37) -> (-35.3701, -35)
  line L591 (-31.04, -37.5) -> (-33.3494, -37.5)
  line L592 (-33.3494, -37.5) -> (-34.2154, -39)
  line L593 (-30.1739, -39) -> (-31.04, -37.5)
  line L594 (-52.6906, -30) -> (-55, -30)
  line L595 (-55, -30) -> (-56, -31.7321)
  line L596 (-56, -32.2679) -> (-55, -34)
  line L597 (-55, -34) -> (-52.6906, -34)
  line L598 (-52.6906, -34) -> (-51.5359, -32)
  line L599 (-51.5359, -32) -> (-52.6906, -30)
  line L600 (-48.3605, -32.5) -> (-50.6699, -32.5)
  line L601 (-50.6699, -32.5) -> (-51.8246, -34.5)
  line L602 (-51.8246, -34.5) -> (-50.6699, -36.5)
  line L603 (-50.6699, -36.5) -> (-48.3605, -36.5)
  line L604 (-48.3605, -36.5) -> (-47.2058, -34.5)
  line L605 (-47.2058, -34.5) -> (-48.3605, -32.5)
  line L606 (-44.0303, -35) -> (-46.3397, -35)
  line L607 (-46.3397, -35) -> (-47.4944, -37)
  line L608 (-47.4944, -37) -> (-46.3397, -39)
  line L609 (-46.3397, -39) -> (-44.0303, -39)
  line L610 (-44.0303, -39) -> (-42.8756, -37)
  line L611 (-42.8756, -37) -> (-44.0303, -35)
  line L612 (-39.7002, -37.5) -> (-42.0096, -37.5)
  line L613 (-42.0096, -37.5) -> (-42.8756, -39)
  line L614 (-38.8342, -39) -> (-39.7002, -37.5)
  line L615 (-52.6906, -35) -> (-55, -35)
  line L616 (-55, -35) -> (-56, -36.7321)
  line L617 (-56, -37.2679) -> (-55, -39)
  line L618 (-55, -39) -> (-52.6906, -39)
  line L619 (-52.6906, -39) -> (-51.5359, -37)
  line L620 (-51.5359, -37) -> (-52.6906, -35)
  line L621 (-48.3605, -37.5) -> (-50.6699, -37.5)
  line L622 (-50.6699, -37.5) -> (-51.5359, -39)
  line L623 (-47.4944, -39) -> (-48.3605, -37.5)
  line L624 (-56, -2.2679) -> (-56, -1.7321)
  line L625 (-55, 0) -> (-52.6906, 0)
  line L626 (-51.5359, 0) -> (-47.4944, 0)
  line L627 (-46.3397, 0) -> (-44.0303, 0)
  line L628 (-42.8756, 0) -> (-38.8342, 0)
  line L629 (-37.6795, 0) -> (-35.3701, 0)
  line L630 (-34.2154, 0) -> (-30.1739, 0)
  line L631 (-29.0192, 0) -> (-26.7098, 0)
  line L632 (-25.5551, 0) -> (-21.5137, 0)
  line L633 (-20.359, 0) -> (-18.0496, 0)
  line L634 (-16.8949, 0) -> (-12.8534, 0)
  line L635 (-11.6987, 0) -> (-9.3893, 0)
  line L636 (-8.2346, 0) -> (-4.1932, 0)
  line L637 (-3.0385, 0) -> (-0.7291, 0)
  line L638 (0, -1.2628) -> (0, -2.7372)
  line L639 (0, -6.2628) -> (0, -7.7372)
  line L640 (0, -11.2628) -> (0, -12.7372)
  line L641 (0, -16.2628) -> (0, -17.7372)
  line L642 (0, -21.2628) -> (0, -22.7372)
  line L643 (0, -26.2628) -> (0, -27.7372)
  line L644 (0, -31.2628) -> (0, -32.7372)
  line L645 (0, -36.2628) -> (0, -37.7372)
  line L646 (-0.7291, -39) -> (-3.0385, -39)
  line L647 (-4.1932, -39) -> (-8.2346, -39)
  line L648 (-9.3893, -39) -> (-11.6987, -39)
  line L649 (-12.8534, -39) -> (-16.8949, -39)
  line L650 (-18.0496, -39) -> (-20.359, -39)
  line L651 (-21.5137, -39) -> (-25.5551, -39)
  line L652 (-26.7098, -39) -> (-29.0192, -39)
  line L653 (-30.1739, -39) -> (-34.2154, -39)
  line L654 (-35.3701, -39) -> (-37.6795, -39)
  line L655 (-38.8342, -39) -> (-46.3397, -39)
  line L656 (-47.4944, -39) -> (-51.5359, -39)
  line L657 (-52.6906, -39) -> (-55, -39)
  line L658 (-56, -37.2679) -> (-56, -36.7321)
  line L659 (-56, -32.2679) -> (-56, -31.7321)
  line L660 (-56, -27.2679) -> (-56, -26.7321)
  line L661 (-56, -22.2679) -> (-56, -21.7321)
  line L662 (-56, -17.2679) -> (-56, -16.7321)
  line L663 (-56, -12.2679) -> (-56, -11.7321)
  line L664 (-56, -7.2679) -> (-56, -6.7321)
  constraint horizontal L625
  constraint vertical L638
  constraint horizontal L646
  constraint vertical L658
  constraint coincident L167.end L625
  constraint coincident L165.start L625
  constraint coincident L110.end L625
  constraint coincident L108.start L625
  constraint coincident L65.end L625
  constraint coincident L63.start L625
  constraint coincident L30.start L625
  constraint coincident L32.end L625
  constraint collinear L624 L658
  constraint collinear L625 L626
  constraint collinear L626 L627
  constraint collinear L627 L628
  constraint collinear L628 L629
  constraint collinear L629 L630
  constraint collinear L630 L631
  constraint collinear L631 L632
  constraint collinear L632 L633
  constraint coincident L9.start L633
  constraint collinear L633 L635
  constraint collinear L633 L634
  constraint coincident L0.start L635
  constraint coincident L2.end L635
  constraint collinear L635 L636
  constraint collinear L636 L637
  constraint collinear L638 L639
  constraint collinear L639 L640
  constraint collinear L640 L641
  constraint collinear L641 L642
  constraint collinear L642 L643
  constraint collinear L643 L644
  constraint collinear L644 L645
  constraint coincident L458.start L646
  constraint collinear L646 L647
  constraint collinear L647 L648
  constraint collinear L648 L649
  constraint collinear L649 L650
  constraint collinear L650 L651
  constraint collinear L651 L652
  constraint coincident L593.start L652
  constraint collinear L652 L653
  constraint collinear L653 L654
  constraint coincident L614.start L654
  constraint collinear L654 L655
  constraint coincident L613.end L655
  constraint collinear L655 L656
  constraint collinear L656 L657
  constraint collinear L658 L659
  constraint collinear L659 L660
  constraint collinear L660 L661
  constraint collinear L661 L662
  constraint collinear L662 L663
  constraint collinear L663 L664
sketch "Sketch6" plane through (57, 0, 0) normal (-1, 0, 0) x (0, -1, 0)
  circle A0 centre (-27, 12.5) radius 5
  line L0 (-40, 3) -> (1, 3)
  line L1 (1, 3) -> (1, 21)
  line L2 (1, 21) -> (-40, 21)
  line L3 (-40, 21) -> (-40, 3)
  line L4 (-25.8, 7) -> (-28.3, 7)
  line L5 (-28.3, 7) -> (-28.3, 4)
  line L6 (-28.3, 4) -> (-25.8, 4)
  line L7 (-25.8, 4) -> (-25.8, 7)
  constraint horizontal L4
  constraint vertical L5
  constraint horizontal L6
  constraint vertical L7
extrude "Extrude7" cut sketch "Sketch6" against normal blind 1 contours L4 L5 L6 L7
sketch "Sketch7" plane through (0, 0, 3) normal (0, 0, 1) x (-1, 0, 0)
  line L0 (1, 1) -> (-57, 1)
  line L1 (-57, 1) -> (-57, -40)
  line L2 (-57, -40) -> (1, -40)
  line L3 (1, -40) -> (1, 1)
  line L4 (-57, 1) -> (-50, 1)
  line L5 (-50, 1) -> (-50, -6)
  line L6 (-50, -6) -> (-57, -6)
  line L7 (-57, -6) -> (-57, 1)
  line L8 (-57, -40) -> (-50, -40)
  line L9 (-50, -40) -> (-50, -33)
  line L10 (-50, -33) -> (-57, -33)
  line L11 (-57, -33) -> (-57, -40)
  line L12 (1, -40) -> (-5, -40)
  line L13 (-5, -40) -> (-5, -35)
  line L14 (-5, -35) -> (1, -35)
  line L15 (1, -35) -> (1, -40)
  line L16 (1, 1) -> (-5, 1)
  line L17 (-5, 1) -> (-5, -4)
  line L18 (-5, -4) -> (1, -4)
  line L19 (1, -4) -> (1, 1)
  circle A0 centre (-52.5, -2) radius 1.5
  circle A1 centre (-52.5, -37) radius 1.5
  dimension "d23" = 4.5
  dimension "d24" = 3
  dimension "d25" = 3
  constraint horizontal L4
  constraint vertical L5
  constraint horizontal L6
  constraint vertical L7
  constraint coincident L0.end L1.start
  constraint horizontal L8
  constraint vertical L9
  constraint horizontal L10
  constraint vertical L11
  constraint coincident L1.end L2.start
  constraint horizontal L12
  constraint vertical L13
  constraint horizontal L14
  constraint vertical L15
  constraint coincident L2.end L3.start
  constraint horizontal L16
  constraint vertical L17
  constraint horizontal L18
  constraint vertical L19
  constraint coincident L0.start L3.end
  measures "d23" distance of L7 A0.centre
  measures "d24" distance of L4 A0.centre
  measures "d25" distance of L8 A1.centre
extrude "Extrude8" add sketch "Sketch7" along normal blind 2 contours L0 L3 L16 L17 L18 L19 | L0 L1 L4 L5 L6 L7 | L2 L3 L12 L13 L14 L15 | L1 L2 L8 L9 L10 L11
sketch "Sketch8" plane through (0, 0, 3) normal (0, 0, 1) x (-1, 0, 0)
  line L0 (-48.7321, -5.5) -> (-47, -8.5)
  line L1 (-47, -8.5) -> (-43.5359, -8.5)
  line L2 (-43.5359, -8.5) -> (-41.8038, -5.5)
  line L3 (-41.8038, -5.5) -> (-43.5359, -2.5)
  line L4 (-43.5359, -2.5) -> (-47, -2.5)
  line L5 (-47, -2.5) -> (-48.7321, -5.5)
  line L6 (-48.7321, -12.5) -> (-47, -15.5)
  line L7 (-47, -15.5) -> (-43.5359, -15.5)
  line L8 (-43.5359, -15.5) -> (-41.8038, -12.5)
  line L9 (-41.8038, -12.5) -> (-43.5359, -9.5)
  line L10 (-43.5359, -9.5) -> (-47, -9.5)
  line L11 (-47, -9.5) -> (-48.7321, -12.5)
  line L12 (-48.7321, -19.5) -> (-47, -22.5)
  line L13 (-47, -22.5) -> (-43.5359, -22.5)
  line L14 (-43.5359, -22.5) -> (-41.8038, -19.5)
  line L15 (-41.8038, -19.5) -> (-43.5359, -16.5)
  line L16 (-43.5359, -16.5) -> (-47, -16.5)
  line L17 (-47, -16.5) -> (-48.7321, -19.5)
  line L18 (-48.7321, -26.5) -> (-47, -29.5)
  line L19 (-47, -29.5) -> (-43.5359, -29.5)
  line L20 (-43.5359, -29.5) -> (-41.8038, -26.5)
  line L21 (-41.8038, -26.5) -> (-43.5359, -23.5)
  line L22 (-43.5359, -23.5) -> (-47, -23.5)
  line L23 (-47, -23.5) -> (-48.7321, -26.5)
  line L24 (-48.7321, -33.5) -> (-47, -36.5)
  line L25 (-47, -36.5) -> (-43.5359, -36.5)
  line L26 (-43.5359, -36.5) -> (-41.8038, -33.5)
  line L27 (-41.8038, -33.5) -> (-43.5359, -30.5)
  line L28 (-43.5359, -30.5) -> (-47, -30.5)
  line L29 (-47, -30.5) -> (-48.7321, -33.5)
  line L30 (-42.6699, -9) -> (-40.9378, -12)
  line L31 (-40.9378, -12) -> (-37.4737, -12)
  line L32 (-37.4737, -12) -> (-35.7417, -9)
  line L33 (-35.7417, -9) -> (-37.4737, -6)
  line L34 (-37.4737, -6) -> (-40.9378, -6)
  line L35 (-40.9378, -6) -> (-42.6699, -9)
  line L36 (-42.6699, -16) -> (-40.9378, -19)
  line L37 (-40.9378, -19) -> (-37.4737, -19)
  line L38 (-37.4737, -19) -> (-35.7417, -16)
  line L39 (-35.7417, -16) -> (-37.4737, -13)
  line L40 (-37.4737, -13) -> (-40.9378, -13)
  line L41 (-40.9378, -13) -> (-42.6699, -16)
  line L42 (-42.6699, -23) -> (-40.9378, -26)
  line L43 (-40.9378, -26) -> (-37.4737, -26)
  line L44 (-37.4737, -26) -> (-35.7417, -23)
  line L45 (-35.7417, -23) -> (-37.4737, -20)
  line L46 (-37.4737, -20) -> (-40.9378, -20)
  line L47 (-40.9378, -20) -> (-42.6699, -23)
  line L48 (-42.6699, -30) -> (-40.9378, -33)
  line L49 (-40.9378, -33) -> (-37.4737, -33)
  line L50 (-37.4737, -33) -> (-35.7417, -30)
  line L51 (-35.7417, -30) -> (-37.4737, -27)
  line L52 (-37.4737, -27) -> (-40.9378, -27)
  line L53 (-40.9378, -27) -> (-42.6699, -30)
  line L54 (-36.6077, -5.5) -> (-34.8756, -8.5)
  line L55 (-34.8756, -8.5) -> (-31.4115, -8.5)
  line L56 (-31.4115, -8.5) -> (-29.6795, -5.5)
  line L57 (-29.6795, -5.5) -> (-31.4115, -2.5)
  line L58 (-31.4115, -2.5) -> (-34.8756, -2.5)
  line L59 (-34.8756, -2.5) -> (-36.6077, -5.5)
  line L60 (-36.6077, -12.5) -> (-34.8756, -15.5)
  line L61 (-34.8756, -15.5) -> (-31.4115, -15.5)
  line L62 (-31.4115, -15.5) -> (-29.6795, -12.5)
  line L63 (-29.6795, -12.5) -> (-31.4115, -9.5)
  line L64 (-31.4115, -9.5) -> (-34.8756, -9.5)
  line L65 (-34.8756, -9.5) -> (-36.6077, -12.5)
  line L66 (-36.6077, -19.5) -> (-34.8756, -22.5)
  line L67 (-34.8756, -22.5) -> (-31.4115, -22.5)
  line L68 (-31.4115, -22.5) -> (-29.6795, -19.5)
  line L69 (-29.6795, -19.5) -> (-31.4115, -16.5)
  line L70 (-31.4115, -16.5) -> (-34.8756, -16.5)
  line L71 (-34.8756, -16.5) -> (-36.6077, -19.5)
  line L72 (-36.6077, -26.5) -> (-34.8756, -29.5)
  line L73 (-34.8756, -29.5) -> (-31.4115, -29.5)
  line L74 (-31.4115, -29.5) -> (-29.6795, -26.5)
  line L75 (-29.6795, -26.5) -> (-31.4115, -23.5)
  line L76 (-31.4115, -23.5) -> (-34.8756, -23.5)
  line L77 (-34.8756, -23.5) -> (-36.6077, -26.5)
  line L78 (-36.6077, -33.5) -> (-34.8756, -36.5)
  line L79 (-34.8756, -36.5) -> (-31.4115, -36.5)
  line L80 (-31.4115, -36.5) -> (-29.6795, -33.5)
  line L81 (-29.6795, -33.5) -> (-31.4115, -30.5)
  line L82 (-31.4115, -30.5) -> (-34.8756, -30.5)
  line L83 (-34.8756, -30.5) -> (-36.6077, -33.5)
  line L84 (-30.5455, -9) -> (-28.8135, -12)
  line L85 (-28.8135, -12) -> (-25.3494, -12)
  line L86 (-25.3494, -12) -> (-23.6173, -9)
  line L87 (-23.6173, -9) -> (-25.3494, -6)
  line L88 (-25.3494, -6) -> (-28.8135, -6)
  line L89 (-28.8135, -6) -> (-30.5455, -9)
  line L90 (-30.5455, -16) -> (-28.8135, -19)
  line L91 (-28.8135, -19) -> (-25.3494, -19)
  line L92 (-25.3494, -19) -> (-23.6173, -16)
  line L93 (-23.6173, -16) -> (-25.3494, -13)
  line L94 (-25.3494, -13) -> (-28.8135, -13)
  line L95 (-28.8135, -13) -> (-30.5455, -16)
  line L96 (-30.5455, -23) -> (-28.8135, -26)
  line L97 (-28.8135, -26) -> (-25.3494, -26)
  line L98 (-25.3494, -26) -> (-23.6173, -23)
  line L99 (-23.6173, -23) -> (-25.3494, -20)
  line L100 (-25.3494, -20) -> (-28.8135, -20)
  line L101 (-28.8135, -20) -> (-30.5455, -23)
  line L102 (-30.5455, -30) -> (-28.8135, -33)
  line L103 (-28.8135, -33) -> (-25.3494, -33)
  line L104 (-25.3494, -33) -> (-23.6173, -30)
  line L105 (-23.6173, -30) -> (-25.3494, -27)
  line L106 (-25.3494, -27) -> (-28.8135, -27)
  line L107 (-28.8135, -27) -> (-30.5455, -30)
  line L108 (-24.4833, -5.5) -> (-22.7513, -8.5)
  line L109 (-22.7513, -8.5) -> (-19.2872, -8.5)
  line L110 (-19.2872, -8.5) -> (-17.5551, -5.5)
  line L111 (-17.5551, -5.5) -> (-19.2872, -2.5)
  line L112 (-19.2872, -2.5) -> (-22.7513, -2.5)
  line L113 (-22.7513, -2.5) -> (-24.4833, -5.5)
  line L114 (-24.4833, -12.5) -> (-22.7513, -15.5)
  line L115 (-22.7513, -15.5) -> (-19.2872, -15.5)
  line L116 (-19.2872, -15.5) -> (-17.5551, -12.5)
  line L117 (-17.5551, -12.5) -> (-19.2872, -9.5)
  line L118 (-19.2872, -9.5) -> (-22.7513, -9.5)
  line L119 (-22.7513, -9.5) -> (-24.4833, -12.5)
  line L120 (-24.4833, -19.5) -> (-22.7513, -22.5)
  line L121 (-22.7513, -22.5) -> (-19.2872, -22.5)
  line L122 (-19.2872, -22.5) -> (-17.5551, -19.5)
  line L123 (-17.5551, -19.5) -> (-19.2872, -16.5)
  line L124 (-19.2872, -16.5) -> (-22.7513, -16.5)
  line L125 (-22.7513, -16.5) -> (-24.4833, -19.5)
  line L126 (-24.4833, -26.5) -> (-22.7513, -29.5)
  line L127 (-22.7513, -29.5) -> (-19.2872, -29.5)
  line L128 (-19.2872, -29.5) -> (-17.5551, -26.5)
  line L129 (-17.5551, -26.5) -> (-19.2872, -23.5)
  line L130 (-19.2872, -23.5) -> (-22.7513, -23.5)
  line L131 (-22.7513, -23.5) -> (-24.4833, -26.5)
  line L132 (-24.4833, -33.5) -> (-22.7513, -36.5)
  line L133 (-22.7513, -36.5) -> (-19.2872, -36.5)
  line L134 (-19.2872, -36.5) -> (-17.5551, -33.5)
  line L135 (-17.5551, -33.5) -> (-19.2872, -30.5)
  line L136 (-19.2872, -30.5) -> (-22.7513, -30.5)
  line L137 (-22.7513, -30.5) -> (-24.4833, -33.5)
  line L138 (-18.4212, -9) -> (-16.6891, -12)
  line L139 (-16.6891, -12) -> (-13.225, -12)
  line L140 (-13.225, -12) -> (-11.493, -9)
  line L141 (-11.493, -9) -> (-13.225, -6)
  line L142 (-13.225, -6) -> (-16.6891, -6)
  line L143 (-16.6891, -6) -> (-18.4212, -9)
  line L144 (-18.4212, -16) -> (-16.6891, -19)
  line L145 (-16.6891, -19) -> (-13.225, -19)
  line L146 (-13.225, -19) -> (-11.493, -16)
  line L147 (-11.493, -16) -> (-13.225, -13)
  line L148 (-13.225, -13) -> (-16.6891, -13)
  line L149 (-16.6891, -13) -> (-18.4212, -16)
  line L150 (-18.4212, -23) -> (-16.6891, -26)
  line L151 (-16.6891, -26) -> (-13.225, -26)
  line L152 (-13.225, -26) -> (-11.493, -23)
  line L153 (-11.493, -23) -> (-13.225, -20)
  line L154 (-13.225, -20) -> (-16.6891, -20)
  line L155 (-16.6891, -20) -> (-18.4212, -23)
  line L156 (-18.4212, -30) -> (-16.6891, -33)
  line L157 (-16.6891, -33) -> (-13.225, -33)
  line L158 (-13.225, -33) -> (-11.493, -30)
  line L159 (-11.493, -30) -> (-13.225, -27)
  line L160 (-13.225, -27) -> (-16.6891, -27)
  line L161 (-16.6891, -27) -> (-18.4212, -30)
  line L162 (-12.359, -5.5) -> (-10.6269, -8.5)
  line L163 (-10.6269, -8.5) -> (-7.1628, -8.5)
  line L164 (-7.1628, -8.5) -> (-5.4308, -5.5)
  line L165 (-5.4308, -5.5) -> (-7.1628, -2.5)
  line L166 (-7.1628, -2.5) -> (-10.6269, -2.5)
  line L167 (-10.6269, -2.5) -> (-12.359, -5.5)
  line L168 (-12.359, -12.5) -> (-10.6269, -15.5)
  line L169 (-10.6269, -15.5) -> (-7.1628, -15.5)
  line L170 (-7.1628, -15.5) -> (-5.4308, -12.5)
  line L171 (-5.4308, -12.5) -> (-7.1628, -9.5)
  line L172 (-7.1628, -9.5) -> (-10.6269, -9.5)
  line L173 (-10.6269, -9.5) -> (-12.359, -12.5)
  line L174 (-12.359, -19.5) -> (-10.6269, -22.5)
  line L175 (-10.6269, -22.5) -> (-7.1628, -22.5)
  line L176 (-7.1628, -22.5) -> (-5.4308, -19.5)
  line L177 (-5.4308, -19.5) -> (-7.1628, -16.5)
  line L178 (-7.1628, -16.5) -> (-10.6269, -16.5)
  line L179 (-10.6269, -16.5) -> (-12.359, -19.5)
  line L180 (-12.359, -26.5) -> (-10.6269, -29.5)
  line L181 (-10.6269, -29.5) -> (-7.1628, -29.5)
  line L182 (-7.1628, -29.5) -> (-5.4308, -26.5)
  line L183 (-5.4308, -26.5) -> (-7.1628, -23.5)
  line L184 (-7.1628, -23.5) -> (-10.6269, -23.5)
  line L185 (-10.6269, -23.5) -> (-12.359, -26.5)
  line L186 (-12.359, -33.5) -> (-10.6269, -36.5)
  line L187 (-10.6269, -36.5) -> (-7.1628, -36.5)
  line L188 (-7.1628, -36.5) -> (-5.4308, -33.5)
  line L189 (-5.4308, -33.5) -> (-7.1628, -30.5)
  line L190 (-7.1628, -30.5) -> (-10.6269, -30.5)
  line L191 (-10.6269, -30.5) -> (-12.359, -33.5)
extrude "Extrude9" cut sketch "Sketch8" against normal blind 3
extrude "Extrude10" cut 4 faces at (55.9944, 36.5921, 5) (3, 36.6667, 5) (55.9944, 2.4079, 5) (3, 0.6667, 5) along direction (0, 0, -1) blind 2
extrude "Extrude11" cut 1 faces at (18.6667, -1.6667, 21) along direction (0, 0, -1) blind 19
extrude "Extrude12" cut 1 faces at (-1.6667, 13.6667, 7) along direction (0, 0, -1) blind 4